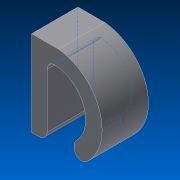
# Autodesk Inventor part: cable hook 5mm
Saved by Autodesk Inventor 2015 (Build 190159000, 159)
## iProperties
Created: 2017-03-25
Part Number: cable hook 5mm
Material: Generic
Document SubType Name: Modeling
Designer: ZigZagJoe
Density: 1 g/cm^3
Appearance: Default
Author: ZigZagJoe
Autodesk Inventor part; units mm, degrees
ref_plane "YZ Plane" through (0, 0, 0) normal (1, 0, 0) x (0, 1, 0)
ref_plane "XZ Plane" through (0, 0, 0) normal (0, 1, 0) x (-1, 0, 0)
ref_plane "XY Plane" through (0, 0, 0) normal (0, 0, 1) x (1, 0, 0)
sketch "Sketch1" plane through (0, 0, 0) normal (0, 1, 0) x (-1, 0, 0)
  line L0 (4.9837, 0.8124) -> (4.9837, -5.2521)
  line L1 (5.9837, -6.2521) -> (6.9837, -6.2521)
  line L2 (6.9837, -6.2521) -> (6.9837, 4.8124)
  line L3 (6.9837, 4.8124) -> (3.5054, 4.8124)
  arc A0 (3.5054, 4.8124) -> (-0.2058, -5.9241) centre (4.0987, -1.4023) ccw
  arc A1 (4.1372, 2.8124) -> (1.1926, -4.2705) centre (4.1372, -1.3411) ccw
  line L4 (1.4837, -4.9758) -> (1.4837, -5.1998)
  arc A2 (1.4837, -4.9758) -> (1.1926, -4.2705) centre (0.4837, -4.9758) ccw
  arc A3 (-0.2058, -5.9241) -> (1.4837, -5.1998) centre (0.4837, -5.1998) ccw
  arc A4 (4.9837, -5.2521) -> (5.9837, -6.2521) centre (5.9837, -5.2521) ccw
  line L5 (4.9837, 0.8124) -> (4.9837, 1.8124)
  line L6 (3.9837, 2.8124) -> (4.1372, 2.8124)
  arc A5 (4.9837, 1.8124) -> (3.9837, 2.8124) centre (3.9837, 1.8124) ccw
  point P0 (0, 0)
  point P1 (4.9837, -6.2521)
  point P2 (1.4837, -7.0713)
  point P3 (1.4837, -4.5365)
  point P4 (4.0342, 2.8111)
  dimension "d1" = 2
  dimension "d5" = 1
  dimension "d6" = 3.5
  dimension "d7" = 5
  dimension "d8" = 1
  dimension "d9" = 2
  dimension "d10" = 1
  constraints: 17 point on circle, 14 end point, 8 tangent, 6 centre point, 4 perpendicular, 4 point on line, 3 vertical, 1 equal radius
  measures "d1" distance of point (4.984, -6.252) L1.end
  measures "d5" radius of A2
  measures "d6" distance from line of L0 L4.end
  measures "d8" radius of A4
  measures "d9" distance between parallel lines of L3 L6
  measures "d10" radius of A5
extrude "Extrusion1" add sketch "Sketch1" along normal blind 6
body "Solid1"
